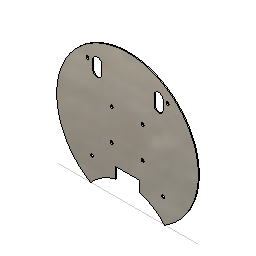
BaseChapaCima+Draw (Autodesk Fusion 360 archive; units mm, degrees)
design "BaseChapaCima"
Autodesk Fusion 360 part; units mm, degrees
sketch "Sketch1" plane through (0, 0, 0) normal (0, 1, 0) x (1, 0, 0)
  circle A0 centre (0, 0) radius 240
  line L0 (0, -240) -> (125, -240)
  line L1 (125, -240) -> (125, -204.878)
  line L2 (0, 240) -> (0, -147)
  line L3 (125, -204.878) -> (-125, -204.878)
  arc A1 (125, -204.878) -> (-125, -204.878) centre (0, -310.9212) ccw
  circle A2 centre (-53.8749, 53.8749) radius 5
  line L4 (-53.8749, 53.8749) -> (51.1251, 53.8749)
  line L5 (51.1251, 53.8749) -> (51.1251, -51.1251)
  line L6 (51.1251, -51.1251) -> (-53.8749, -51.1251)
  line L7 (-53.8749, -51.1251) -> (-53.8749, 53.8749)
  circle A3 centre (51.1251, 53.8749) radius 5
  circle A4 centre (51.1251, -51.1251) radius 5
  circle A5 centre (-53.8749, -51.1251) radius 5
  line L8 (0, 240) -> (250, 240)
  line L9 (-53.8749, 53.8749) -> (-53.8749, 233.8749)
  line L10 (-53.8749, 53.8749) -> (-233.8749, 53.8749)
  line L11 (105.2845, 215.6738) -> (105.2845, 175.6738)
  line L12 (105.2845, 175.6738) -> (105.2845, 115.6738)
  line L13 (105.2845, 115.6738) -> (210.2845, 115.6738)
  line L14 (105.2845, 115.6738) -> (105.2845, 130.6738)
  line L15 (105.2845, 175.6738) -> (105.2845, 160.6738)
  line L16 (120.2845, 130.6738) -> (120.2845, 160.6738)
  arc A6 (120.2845, 160.6738) -> (90.2845, 160.6738) centre (105.2845, 160.6738) ccw
  line L17 (90.2845, 160.6738) -> (90.2845, 130.6738)
  arc A7 (90.2845, 130.6738) -> (120.2845, 130.6738) centre (105.2845, 130.6738) ccw
  line L18 (105.2845, 130.6738) -> (105.2845, 160.6738) construction
  line L19 (0, -147) -> (40, -147)
  line L20 (40, -147) -> (40, -151.9553)
  line L21 (0, -147) -> (0, -115)
  line L22 (0, -115) -> (-40, -115)
  line L23 (40, -151.9553) -> (-40, -151.9553)
  line L24 (-40, -151.9553) -> (-40, -115)
  line L25 (-40, -115) -> (40, -115)
  line L26 (40, -115) -> (40, -151.9553)
  line L27 (-135.688, 197.9615) -> (-135.688, 157.9615)
  line L28 (-135.688, 157.9615) -> (-180.688, 157.9615)
  circle A8 centre (-135.688, 157.9615) radius 5
  line L29 (-135.688, 157.9615) -> (-102.688, 157.9615)
  line L30 (105.2845, 160.6738) -> (-102.688, 160.6738)
  line L31 (-102.688, 160.6738) -> (-102.688, 130.6738)
  line L32 (-117.688, 160.6738) -> (-117.688, 130.6738)
  arc A9 (-117.688, 130.6738) -> (-87.688, 130.6738) centre (-102.688, 130.6738) ccw
  line L33 (-87.688, 130.6738) -> (-87.688, 160.6738)
  arc A10 (-87.688, 160.6738) -> (-117.688, 160.6738) centre (-102.688, 160.6738) ccw
  line L34 (-102.688, 160.6738) -> (-102.688, 130.6738) construction
  line L35 (-102.688, 157.9615) -> (-102.688, 160.6738)
  line L36 (-120.6537, -115) -> (-120.8737, -122.997)
  circle A11 centre (-120.8737, -122.997) radius 5
  line L37 (-40, -115) -> (-210.6537, -115)
  line L38 (-210.6537, -115) -> (-120.6537, -115)
  circle A12 centre (120.8737, -122.997) radius 5
  line L39 (152.5158, 185.3077) -> (67.5158, 185.3077)
  line L40 (67.5158, 185.3077) -> (67.5158, 230.3077)
  circle A13 centre (135.688, 157.9615) radius 5
  dimension "d1" = 480
  dimension "d2" = 125
  dimension "d3" = 387
  dimension "d7" = 10
  dimension "d8" = 105
  dimension "d9" = 105
  dimension "d10" = 10
  dimension "d11" = 10
  dimension "d12" = 10
  dimension "d13" = 250
  dimension "d14" = 180
  dimension "d15" = 180
  dimension "d16" = 40
  dimension "d17" = 60
  dimension "d18" = 105
  dimension "d19" = 15
  dimension "d20" = 15
  dimension "d21" = 30
  dimension "d22" = 40
  dimension "d23" = 32
  dimension "d24" = 40
  dimension "d25" = 40
  dimension "d26" = 45
  dimension "d27" = 10
  dimension "d28" = 33
  dimension "d29" = 30
  dimension "d30" = 30
  dimension "d32" = 8
  dimension "d33" = 10
  dimension "d34" = 90
  dimension "d35" = 85
  dimension "d36" = 45
  constraint coincident A0.centre origin
  constraint coincident A0 L0.start
  constraint horizontal L0
  constraint coincident A0 L1.end
  constraint perpendicular L0 L1
  constraint coincident A0 L2.start
  constraint vertical L2
  constraint coincident A0 L3.end
  constraint perpendicular L1 L3
  constraint coincident L2.end A1
  constraint horizontal L4
  constraint vertical L5
  constraint horizontal L6
  constraint vertical L7
  constraint coincident A2.centre L4.start
  constraint coincident L4.end L5.start
  constraint coincident L5.end L6.start
  constraint coincident L6.end L7.start
  constraint perpendicular L2 L8
  constraint coincident A0 L9.end
  constraint parallel L7 L9
  constraint coincident A0 L10.end
  constraint perpendicular L9 L10
  constraint coincident A0 L11.start
  constraint vertical L11
  constraint parallel L11 L12
  constraint perpendicular L12 L13
  constraint coincident A0 L13.end
  constraint perpendicular L13 L14
  constraint parallel L12 L15
  constraint tangent L16 A6
  constraint tangent A6 L17
  constraint parallel L16 L17
  constraint tangent L17 A7
  constraint tangent L16 A7
  constraint coincident L15.end A6.centre
  constraint parallel L15 L18
  constraint coincident L14.end A7.centre
  constraint perpendicular L2 L19
  constraint coincident A1 L20.end
  constraint perpendicular L19 L20
  constraint perpendicular L19 L21
  constraint perpendicular L2 L22
  constraint horizontal L23
  constraint vertical L24
  constraint horizontal L25
  constraint vertical L26
  constraint coincident A0 L27.start
  constraint parallel L2 L27
  constraint coincident A0 L28.end
  constraint perpendicular L27 L28
  constraint coincident L27.end L28.start
  constraint perpendicular L27 L29
  constraint perpendicular L15 L30
  constraint perpendicular L30 L31
  constraint tangent L32 A9
  constraint tangent A9 L33
  constraint parallel L32 L33
  constraint tangent L33 A10
  constraint tangent L32 A10
  constraint coincident L31.end A9.centre
  constraint perpendicular L29 L34
  constraint coincident L30.end L31.start
  constraint perpendicular L30 L35
  constraint coincident L36.end A11.centre
  constraint coincident A0 L37.end
  constraint perpendicular L24 L37
  constraint parallel L37 L38
  constraint coincident L36.start L38.end
  constraint symmetric L2 A11 A12
  constraint coincident A0 L39.start
  constraint horizontal L39
  constraint coincident A0 L40.end
  constraint perpendicular L39 L40
  constraint symmetric L2 A8 A13
  measures "d1" diameter of A0
  measures "d2" distance of L0.start L0.end
  measures "d3" distance of L2.start L2.end
  measures "d7" diameter of A2
  measures "d8" distance of A2.centre L4.end
  measures "d9" distance of A2.centre L6.end
  measures "d10" diameter of A3
  measures "d11" diameter of A4
  measures "d12" diameter of A5
  measures "d13" distance of L2.start L8.end
  measures "d14" distance of A2.centre L10.end
  measures "d15" distance of A2.centre L9.end
  measures "d16" distance of L11.start L11.end
  measures "d17" distance of L11.end L12.end
  measures "d18" distance of L12.end L13.end
  measures "d19" distance of L12.end L14.end
  measures "d20" distance of L11.end L15.end
  measures "d21" diameter of A6
  measures "d22" distance of L2.end L19.end
  measures "d23" distance of L2.end L21.end
  measures "d24" distance of L21.end L22.end
  measures "d25" distance of L27.start L27.end
  measures "d26" distance of L27.end L28.end
  measures "d27" diameter of A8
  measures "d28" distance of L27.end L29.end
  measures "d29" distance of L30.end L31.end
  measures "d30" diameter of A9
  measures "d32" distance of L36.start L36.end
  measures "d33" diameter of A11
  measures "d34" distance of L37.end L36.start
  measures "d35" distance of L39.start L39.end
  measures "d36" distance of L39.end L40.end
extrude "Extrude1" add sketch "Sketch1" along normal blind 3 contours A0 L2 A1 L4 L5 L6 A3 A4 L13 L17 A7 L20 L25 L26 L30 | A0 L11 L13 L16 A6 A7 L39 | A0 L11 L39 | A0 A1 L24 L37 L38 | A0 L11 L39 L40 | A0 L2 L11 A6 L30 L39 L40 | A0 L2 A2 L6 L7 A5 L10 L22 L25 L37 L38 | A0 A2 L9 L10 L28 A8 L29 L30 L32 A9 L33 | A0 L2 L9 L30 | L2 A2 L4 L9 L30 | A0 L27 L28 A8 | L2 A2 L4 L6 L7 A5 | L2 L4 L5 L6 A3 A4 | A0 L9 L27 A8 L29 L30 L32 A10
move_body "Move1" bodies 1 to x (1, 0, 0) y (0, 0, 1) z (0, -1, 0) at (0, -240, -240)
equation "d2 = ( 250 / 2 ) * 1 mm"
equation "d3 = 355 mm + 32 mm"
